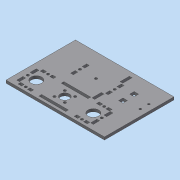
# Autodesk Inventor part: Side
Saved by Autodesk Inventor 2016 SP1 (Build 200210100, 210)
## iProperties
Created: 2016-03-01
Part Number: Side
Material: Generic
Document SubType Name: Modeling
Designer: Mohamed A.
Density: 1 g/cm^3
Appearance: Default
Author: Mohamed A.
Autodesk Inventor part; units mm, degrees
ref_plane "YZ Plane" through (0, 0, 0) normal (1, 0, 0) x (0, 1, 0)
ref_plane "XZ Plane" through (0, 0, 0) normal (0, 1, 0) x (-1, 0, 0)
ref_plane "XY Plane" through (0, 0, 0) normal (0, 0, 1) x (1, 0, 0)
sketch "Sketch1" plane through (0, 0, 0) normal (0, 0, 1) x (1, 0, 0)
  circle A0 centre (0, 0) radius 5.125
  circle A1 centre (32, 0) radius 6
  circle A2 centre (-32, 0) radius 6
  line L0 (-71.1, 0) -> (83.6, 0) construction
  line L1 (-43, 11) -> (61.5, 11)
  line L2 (61.5, 11) -> (61.5, -11)
  line L3 (61.5, -11) -> (-43, -11)
  line L4 (-43, -11) -> (-43, 11)
  line L5 (5.816, 5.816) -> (-5.816, 5.816) construction
  line L6 (-5.816, 5.816) -> (-5.816, -5.816) construction
  line L7 (-5.816, -5.816) -> (5.816, -5.816) construction
  line L8 (5.816, -5.816) -> (5.816, 5.816) construction
  line L9 (5.816, 5.816) -> (-5.816, -5.816) construction
  line L10 (-5.816, 5.816) -> (5.816, -5.816) construction
  circle A3 centre (-5.816, 5.816) radius 1.4
  circle A4 centre (-5.816, -5.816) radius 1.4
  circle A5 centre (5.816, -5.816) radius 1.4
  circle A6 centre (5.816, 5.816) radius 1.4
  line L11 (0, -32.6) -> (0, 76.6) construction
  line L12 (61.5, 11) -> (61.5, 14)
  line L13 (61.5, 14) -> (-43, 14)
  line L14 (-43, 14) -> (-43, 11)
  line L15 (16.5, 14) -> (16.5, 56)
  line L16 (16.5, 56) -> (-16.5, 56)
  line L17 (-16.5, 56) -> (-16.5, 14)
  line L18 (16.5, 56) -> (61.5, 56)
  line L19 (61.5, 56) -> (61.5, 14)
  line L20 (-16.5, 35) -> (61.5, 35) construction
  line L21 (54.5, 39.7625) -> (54.5, 35) construction
  line L22 (54.5, 35) -> (54.5, 30.2375) construction
  circle A7 centre (54.5, 39.7625) radius 1.15
  circle A8 centre (54.5, 30.2375) radius 1.15
  line L23 (-16.5, 56) -> (-27.5, 56)
  line L24 (-27.5, 56) -> (-27.5, 14)
  line L25 (61.5, 56) -> (61.5, 61)
  line L26 (61.5, 61) -> (-27.5, 61)
  line L27 (-27.5, 61) -> (-27.5, 56)
  line L28 (-43, -11) -> (-49, -11)
  line L29 (-49, -11) -> (-49, 61)
  line L30 (-49, 61) -> (-27.5, 61)
  line L31 (-49, -11) -> (-49, -17)
  line L32 (-49, -17) -> (61.5, -17)
  line L33 (61.5, -17) -> (61.5, -11)
  line L34 (-34.5, -14) -> (-34.5, -11) projected
  line L35 (-38.5, -14) -> (-38.5, -11) projected
  line L36 (-24, -14) -> (-24, -11) projected
  line L37 (-28, -14) -> (-28, -11) projected
  line L38 (28.5, -14) -> (28.5, -11) projected
  line L39 (24.5, -14) -> (24.5, -11) projected
  line L40 (39, -14) -> (39, -11) projected
  line L41 (35, -14) -> (35, -11) projected
  line L42 (35, 11) -> (39, 11) projected
  line L43 (39, 11) -> (39, 14) projected
  line L44 (35, 14) -> (39, 14) projected
  line L45 (35, 11) -> (35, 14) projected
  line L46 (24.5, 11) -> (28.5, 11) projected
  line L47 (28.5, 11) -> (28.5, 14) projected
  line L48 (24.5, 14) -> (28.5, 14) projected
  line L49 (24.5, 11) -> (24.5, 14) projected
  line L50 (-28, 11) -> (-24, 11) projected
  line L51 (-24, 11) -> (-24, 14) projected
  line L52 (-28, 14) -> (-24, 14) projected
  line L53 (-28, 11) -> (-28, 14) projected
  line L54 (-38.5, 11) -> (-34.5, 11) projected
  line L55 (-34.5, 11) -> (-34.5, 14) projected
  line L56 (-38.5, 14) -> (-34.5, 14) projected
  line L57 (-38.5, 11) -> (-38.5, 14) projected
  line L58 (-34.5, 14) -> (-28, 11) construction
  line L59 (-28, 14) -> (-34.5, 11) construction
  line L60 (-28, -11) -> (-34.5, -14) construction
  line L61 (-34.5, -11) -> (-28, -14) construction
  line L62 (28.5, -11) -> (35, -14) construction
  line L63 (35, -11) -> (28.5, -14) construction
  line L64 (35, 14) -> (28.5, 11) construction
  line L65 (28.5, 14) -> (35, 11) construction
  circle A9 centre (-31.25, 12.5) radius 1.4
  circle A10 centre (31.75, 12.5) radius 1.4
  circle A11 centre (31.75, -12.5) radius 1.4
  circle A12 centre (-31.25, -12.5) radius 1.4
  line L66 (19.5, 44) -> (19.5, 38.975) projected
  line L67 (19.5, 38.975) -> (22.5, 38.975) projected
  line L68 (22.5, 44) -> (22.5, 38.975) projected
  line L69 (19.5, 44) -> (22.5, 44) projected
  line L70 (19.5, 31.025) -> (19.5, 26) projected
  line L71 (19.5, 26) -> (22.5, 26) projected
  line L72 (22.5, 31.025) -> (22.5, 26) projected
  line L73 (19.5, 31.025) -> (22.5, 31.025) projected
  line L74 (40, -3.975) -> (40, -11) projected
  line L75 (40, -11) -> (43, -11) projected
  line L76 (43, -3.975) -> (43, -11) projected
  line L77 (40, -3.975) -> (43, -3.975) projected
  line L78 (40, 11) -> (40, 3.975) projected
  line L79 (40, 3.975) -> (43, 3.975) projected
  line L80 (43, 11) -> (43, 3.975) projected
  line L81 (40, 11) -> (43, 11) projected
  line L82 (-43, 11) -> (-43, 3.975) projected
  line L83 (-43, 3.975) -> (-40, 3.975) projected
  line L84 (-40, 11) -> (-40, 3.975) projected
  line L85 (-43, 11) -> (-40, 11) projected
  line L86 (-43, -3.975) -> (-43, -11) projected
  line L87 (-43, -11) -> (-40, -11) projected
  line L88 (-40, -3.975) -> (-40, -11) projected
  line L89 (-43, -3.975) -> (-40, -3.975) projected
  line L90 (16.5, 56) -> (16.5, 45.5) projected
  line L91 (16.5, 45.5) -> (19.5, 45.5) projected
  line L92 (19.5, 56) -> (19.5, 45.5) projected
  line L93 (16.5, 56) -> (19.5, 56) projected
  line L94 (16.5, 24.5) -> (16.5, 14) projected
  line L95 (16.5, 14) -> (19.5, 14) projected
  line L96 (19.5, 24.5) -> (19.5, 14) projected
  line L97 (16.5, 24.5) -> (19.5, 24.5) projected
  line L98 (22.5, 38.975) -> (19.5, 31.025) construction
  line L99 (19.5, 38.975) -> (22.5, 31.025) construction
  line L100 (43, 3.975) -> (40, -3.975) construction
  line L101 (43, -3.975) -> (40, 3.975) construction
  line L102 (-40, 3.975) -> (-43, -3.975) construction
  line L103 (-40, -3.975) -> (-43, 3.975) construction
  circle A13 centre (-41.5, 0) radius 1.4
  circle A14 centre (41.5, 0) radius 1.4
  circle A15 centre (21, 35) radius 1.4
  line L104 (-38.5, -14) -> (-34.5, -14) projected
  line L105 (-38.5, -11) -> (-34.5, -11) projected
  line L106 (35, -14) -> (39, -14) projected
  line L107 (35, -11) -> (39, -11) projected
  line L108 (24.5, -14) -> (28.5, -14) projected
  line L109 (24.5, -11) -> (28.5, -11) projected
  line L110 (-28, -14) -> (-24, -14) projected
  line L111 (-28, -11) -> (-24, -11) projected
  line L112 (15, 11) -> (-15, 11) projected
  line L113 (-15, 11) -> (-15, 14) projected
  line L114 (15, 14) -> (-15, 14) projected
  line L115 (15, 11) -> (15, 14) projected
  line L116 (15, -14) -> (-15, -14) projected
  line L117 (-15, -14) -> (-15, -11) projected
  line L118 (15, -11) -> (-15, -11) projected
  line L119 (15, -14) -> (15, -11) projected
  line L120 (-19.5, 38.975) -> (-19.5, 44) projected
  line L121 (-19.5, 44) -> (-16.5, 44) projected
  line L122 (-16.5, 38.975) -> (-16.5, 44) projected
  line L123 (-19.5, 38.975) -> (-16.5, 38.975) projected
  line L124 (-19.5, 26) -> (-19.5, 31.025) projected
  line L125 (-19.5, 31.025) -> (-16.5, 31.025) projected
  line L126 (-16.5, 26) -> (-16.5, 31.025) projected
  line L127 (-19.5, 26) -> (-16.5, 26) projected
  line L128 (-16.5, 38.975) -> (-19.5, 31.025) construction
  line L129 (-19.5, 38.975) -> (-16.5, 31.025) construction
  circle A16 centre (-18, 35) radius 1.4
  circle A17 centre (0, 35) radius 1.4
  dimension "d0" = 10.25
  dimension "d1" = 12
  dimension "d2" = 12
  dimension "d3" = 32
  dimension "d4" = 32
  dimension "d8" = 11.6319
  dimension "d9" = 11.6319
  dimension "d10" = 2.8
  dimension "d11" = 2.8
  dimension "d12" = 2.8
  dimension "d13" = 2.8
  dimension "d20" = 9.525
  dimension "d21" = 2.3
  dimension "d22" = 2.3
  dimension "d23" = 7
  dimension "d27" = 6
  dimension "d28" = 6
  dimension "d29" = 2.8
  dimension "d30" = 2.8
  dimension "d31" = 2.8
  dimension "d32" = 2.8
  dimension "d33" = 2.8
  dimension "d34" = 2.8
  dimension "d35" = 2.8
  dimension "d49" = 11
  dimension "d50" = 5
  dimension "d51" = 45
  dimension "d52" = 2.8
  dimension "d53" = 2.8
  constraints: 96 end point, 18 centre point, 14 perpendicular, 13 midpoint, 13 parallel, 9 point on line, 7 coincident, 5 vertical, 4 horizontal, 1 collinear, 2 other
  measures "d0" diameter of A0
  measures "d1" diameter of A1
  measures "d2" diameter of A2
  measures "d3" distance of A1.centre point (0, 0)
  measures "d4" distance of point (0, 0) A2.centre
  measures "d8" distance of L5.end L6.end
  measures "d9" distance of L5.start L5.end
  measures "d10" diameter of A3
  measures "d11" diameter of A4
  measures "d12" diameter of A5
  measures "d13" diameter of A6
  measures "d20" distance of L22.end L21.start
  measures "d21" diameter of A7
  measures "d22" diameter of A8
  measures "d23" distance between parallel lines of L19 L21
  measures "d27" distance of L3.end L28.end
  measures "d28" distance of L28.end L31.end
  measures "d29" diameter of A9
  measures "d30" diameter of A10
  measures "d31" diameter of A11
  measures "d32" diameter of A12
  measures "d33" diameter of A13
  measures "d34" diameter of A14
  measures "d35" diameter of A15
  measures "d49" distance between parallel lines of L17 L24
  measures "d50" distance between parallel lines of L18 L26
  measures "d51" distance between parallel lines of L15 L19
  measures "d52" diameter of A16
  measures "d53" diameter of A17
extrude "Extrusion1" add sketch "Sketch1" along normal blind 3 contours L14 L13 L57 L1 | L4 L28 L29 L30 L27 L24 L13 L14 | L1 L78 L79 L80 L2 L3 L76 L77 L74 L88 L89 L4 L83 L84 | L55 L13 L53 L1 | L3 L35 L104 L34 L37 L110 L36 L117 L116 L119 L39 L108 L38 L41 L106 L40 L33 L32 L31 L28 | L51 L13 L113 L1 | L24 L23 L17 L121 L120 L123 L125 L124 L127 L13 | L26 L25 L18 L16 L23 L27 | L115 L13 L49 L1 | L13 L17 L16 L15 | L19 L13 L96 L97 L15 L91 L92 L18 | L1 L43 L13 L12 | L47 L13 L45 L1
sketch "Sketch4" plane through (0, 0, 0) normal (0, 0, -1) x (-1, 0, 0)
  circle A0 centre (-54.5, 39.7625) radius 1.15 projected
  circle A1 centre (-54.5, 30.2375) radius 1.15 projected
  circle A2 centre (-21, 35) radius 1.4 projected
  line L0 (-21, 35) -> (-54.5, 35) construction
  line L1 (-39.0334, 43.7408) -> (-34.0334, 43.7408)
  line L2 (-34.0334, 43.7408) -> (-34.0334, 38.7408)
  line L3 (-34.0334, 38.7408) -> (-39.0334, 38.7408)
  line L4 (-39.0334, 38.7408) -> (-39.0334, 43.7408)
  line L5 (-39.0334, 43.7408) -> (-34.0334, 38.7408) construction
  line L6 (-34.0334, 43.7408) -> (-39.0334, 38.7408) construction
  line L7 (-39.0334, 31.2592) -> (-34.0334, 31.2592)
  line L8 (-34.0334, 31.2592) -> (-34.0334, 26.2592)
  line L9 (-34.0334, 26.2592) -> (-39.0334, 26.2592)
  line L10 (-39.0334, 26.2592) -> (-39.0334, 31.2592)
  line L11 (-39.0334, 31.2592) -> (-34.0334, 26.2592) construction
  line L12 (-34.0334, 31.2592) -> (-39.0334, 26.2592) construction
  line L13 (-36.5334, 41.2408) -> (-36.5334, 35) construction
  line L14 (-36.5334, 35) -> (-36.5334, 28.7592) construction
  point P0 (0, 0)
  dimension "d43" = 5
  dimension "d44" = 5
  dimension "d45" = 5
  dimension "d46" = 5
  constraints: 30 end point, 4 midpoint, 4 parallel, 4 perpendicular, 3 horizontal, 1 collinear, 1 point on line
  measures "d43" distance of L2.end L3.end
  measures "d44" distance of L1.end L2.end
  measures "d45" distance of L8.end L9.end
  measures "d46" distance of L7.end L8.end
extrude "Extrusion3" cut sketch "Sketch4" against normal blind 3 contours L1 L2 L3 L4 | L7 L8 L9 L10
equation "\"d1\" = d2"
body "Solid1"
